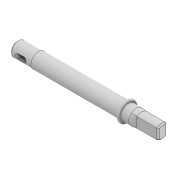
# Autodesk Inventor part: axle
Saved by Autodesk Inventor 2022 (Build 260153000, 153)
## iProperties
Created: 2024-03-20
Part Number: axle
Material: Generic
Document SubType Name: Modeling
Designer: david
Density: 1 g/cm^3
Appearance: Default
Author: david
Autodesk Inventor part; units mm, degrees
ref_plane "YZ Plane" through (0, 0, 0) normal (1, 0, 0) x (0, 1, 0)
ref_plane "XZ Plane" through (0, 0, 0) normal (0, 1, 0) x (-1, 0, 0)
ref_plane "XY Plane" through (0, 0, 0) normal (0, 0, 1) x (1, 0, 0)
sketch "Sketch1" plane through (0, 0, 0) normal (1, 0, 0) x (0, 1, 0)
  circle A0 centre (0, 0) radius 2.85
  dimension "diameter" = 5.7
  constraints: 1 centre point, 1 coincident
  measures "diameter" diameter of A0
extrude "Shaft" add sketch "Sketch1" along normal mid plane 45
sketch "Sketch2" plane through (0, 0, 0) normal (0, 0, 1) x (1, 0, 0)
  line L0 (-22.5, -2.85) -> (-22.5, 2.85) construction
  line L1 (22.5, -2.85) -> (-22.5, -2.85) construction
  line L2 (22.5, 2.85) -> (22.5, -2.85) construction
  line L3 (-22.5, 2.85) -> (22.5, 2.85) construction
  line L4 (-22.5, -2.85) -> (22.5, -2.85) projected
  line L5 (-15.5, -2.85) -> (-15.5, -2.85)
  line L6 (-22.5, -2.85) -> (22.5, -2.85) projected
  line L7 (-20.5, 0) -> (-16.5, 0) construction
  line L8 (-19.6, -0.9) -> (-17.4, -0.9)
  line L9 (-17.4, 0.9) -> (-19.6, 0.9)
  arc A0 (-19.6, 0.9) -> (-19.6, -0.9) centre (-19.6, 0) ccw
  arc A1 (-17.4, -0.9) -> (-17.4, 0.9) centre (-17.4, 0) ccw
  point P0 (0, 0)
  point P1 (22.5, 0)
  point P2 (-18.5, 0)
  dimension "d17" = 1.8
  dimension "d20" = 2
  dimension "d21" = 1
  dimension "d22" = 7
  constraints: 10 end point, 6 point on circle, 4 tangent, 3 point on line, 2 centre point, 2 midpoint, 1 horizontal, 1 horizontal alignment, 1 parallel, 1 perpendicular, 3 other
  measures "d17" distance between parallel lines of L8 L9
  measures "d20" distance from line of L0 L7.start
  measures "d21" distance from line of L5 L7.end
  measures "d22" distance of L0.start L5.start
extrude "Slot" cut sketch "Sketch2" along normal through all both and the other way through all
ref_plane "Work Plane1" through (24.5, 0, 0) normal (1, 0, 0) x (0, 0, -1)
sketch "Sketch3" plane through (24.5, 0, 0) normal (1, 0, 0) x (0, 0, -1)
  arc A0 (-1.8875, 2) -> (-1.8875, -2) centre (0, 0) ccw construction
  line L0 (-1.8875, -2) -> (1.8875, -2) construction
  line L1 (1.8875, -2) -> (1.8875, 2)
  line L2 (1.8875, 2) -> (-1.8875, 2) construction
  line L3 (-1.8875, 2) -> (-1.8875, -2)
  line L4 (-1.8875, -2) -> (1.8875, 2) construction
  line L5 (1.8875, -2) -> (0, 0) construction
  arc A1 (1.8875, 2) -> (-1.8875, 2) centre (0, 0) ccw
  arc A2 (1.8875, -2) -> (1.8875, 2) centre (0, 0) ccw construction
  arc A3 (-1.8875, -2) -> (1.8875, -2) centre (0, 0) ccw
  line L6 (0, 0) -> (-1.8875, 2) construction
  dimension "d23" = 5.5
  dimension "d24" = 4
  constraints: 14 end point, 8 point on circle, 4 centre point, 2 parallel, 1 coincident, 1 horizontal, 1 midpoint, 1 perpendicular
  measures "d23" diameter of A0
  measures "d24" distance of L1.end L0.end
extrude "Wheel Inert Profile" add sketch "Sketch3" along normal blind 8
thicken "Offset for Wheel" operation add thickness 0.15 both sides no extend neighbours yes toward (0, 0, 1) faces at (27.1667, -0.6667, -1.8875) (29.8333, 2.1307, 1.7386) (29.8333, -2.1307, -1.7386) (27.1667, 0.6667, 1.8875)
loft "Loft1" add section 1 edges at (24.5, 2.6, 0) (24.5, 0, -1.7375) (24.5, -2.6, 0) (24.5, 0, 1.7375) section 2 edges at (22.5, -2.85, 0)
ref_plane "Work Plane2" through (18.5, 0, 0) normal (-1, 0, 0) x (0, 0, 1)
sketch "Sketch4" plane through (18.5, 0, 0) normal (-1, 0, 0) x (0, 0, 1)
  circle A0 centre (0, 0) radius 3.75
  dimension "d35" = 7.5
  constraints: 1 centre point, 1 coincident
  measures "d35" diameter of A0
extrude "Stopper" add sketch "Sketch4" against normal blind 1
fillet "Fillet1" radius 0.5 2 edges at (18.5, 0, -3.75) (19.5, 0, -3.75)
sketch "Sketch5" plane through (-22.5, 0, 0) normal (-1, 0, 0) x (0, 0, 1)
  circle A0 centre (0, 0) radius 2.85 projected
  circle A1 centre (0, 0) radius 2.65
  dimension "d48" = 5.3
  constraints: 1 centre point
  measures "d48" diameter of A1
extrude "Offset" [suppressed]
fillet "Fillet2" [suppressed]
chamfer "Chamfer1" [suppressed]
sketch "Sketch6" plane through (-22.5, 0, 0) normal (-1, 0, 0) x (0, 0, 1)
  circle A0 centre (0, 0) radius 2.85 projected
  circle A1 centre (0, 0) radius 2.75 construction
  circle A2 centre (0, 0) radius 2.7
  dimension "d52" = 5.5
  dimension "d53" = 0.05
  constraints: 2 centre point, 1 coincident
  measures "d52" diameter of A1
  measures "d53" radial gap between concentric circles of A1 A2
extrude "Extrusion6" cut sketch "Sketch6" against normal blind 8
chamfer "Chamfer2" distance 0.5 angle 45 5 edges at (32.5, 2.6, 0) (32.5, 0, 1.7375) (32.5, 0, -1.7375) (32.5, -2.6, 0) (-22.5, 0, -2.7)
body "Solid1"
